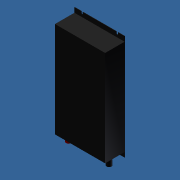
# Autodesk Inventor part: 2kW inverter
Saved by Autodesk Inventor 2012 (Build 160160000, 160)
## iProperties
Created: 2012-06-21
Part Number: 2kW inverter
Material: Default
Document SubType Name: Modeling
Designer: Ed
Density: 0.921071 g/cm^3
Mass: 5600 g
Surface Area: 2636.64 cm^2
Volume: 6079.88 cm^3
Author: Ed
Autodesk Inventor part; units mm, degrees
ref_plane "YZ Plane" through (0, 0, 0) normal (1, 0, 0) x (0, 1, 0)
ref_plane "XZ Plane" through (0, 0, 0) normal (0, 1, 0) x (-1, 0, 0)
ref_plane "XY Plane" through (0, 0, 0) normal (0, 0, 1) x (1, 0, 0)
sketch "Sketch1" plane through (0, 0, 0) normal (0, 0, 1) x (1, 0, 0)
  line L0 (-100.0125, -209.55) -> (100.0125, -209.55)
  line L1 (100.0125, -209.55) -> (100.0125, 209.55)
  line L2 (100.0125, 209.55) -> (-100.0125, 209.55)
  line L3 (-100.0125, 209.55) -> (-100.0125, -209.55)
  circle A0 centre (69.85, 203.2) radius 3.175
  line L4 (66.675, 209.55) -> (73.025, 209.55)
  line L5 (73.025, 209.55) -> (73.025, 203.2)
  line L6 (73.025, 203.2) -> (66.675, 203.2)
  line L7 (66.675, 203.2) -> (66.675, 209.55)
  line L8 (0, 209.55) -> (0, -209.55)
  line L9 (100.0125, 0) -> (-100.0125, 0)
  circle A1 centre (-69.85, 203.2) radius 3.175
  line L10 (-66.675, 209.55) -> (-73.025, 209.55)
  line L11 (-73.025, 209.55) -> (-73.025, 203.2)
  line L12 (-73.025, 203.2) -> (-66.675, 203.2)
  line L13 (-66.675, 203.2) -> (-66.675, 209.55)
  circle A2 centre (69.85, -203.2) radius 3.175
  line L14 (66.675, -209.55) -> (73.025, -209.55)
  line L15 (73.025, -209.55) -> (73.025, -203.2)
  line L16 (73.025, -203.2) -> (66.675, -203.2)
  line L17 (66.675, -203.2) -> (66.675, -209.55)
  circle A3 centre (-69.85, -203.2) radius 3.175
  line L18 (-66.675, -209.55) -> (-73.025, -209.55)
  line L19 (-73.025, -209.55) -> (-73.025, -203.2)
  line L20 (-73.025, -203.2) -> (-66.675, -203.2)
  line L21 (-66.675, -203.2) -> (-66.675, -209.55)
  point P0 (0, 0)
  point P1 (0, 0)
  dimension "d0" = 419.1
  dimension "d1" = 200.025
  dimension "d2" = 6.35
  dimension "d3" = 6.35
  dimension "d4" = 30.1625
  constraints: 44 end point, 18 symmetric about line, 8 point on circle, 6 midpoint, 5 coincident, 4 centre point, 4 parallel, 2 horizontal, 2 perpendicular, 1 point on line, 3 other
  measures "d0" distance of L2.end L0.start
  measures "d1" distance of L0.start L0.end
  measures "d2" diameter of A0
  measures "d3" distance of L4.end L5.end
  measures "d4" distance from line of L1 A0.centre
extrude "Extrusion1" add sketch "Sketch1" along normal blind 1.5875 contours L3 L9 L8 L0 L21 A3 L19 | L3 L2 L11 A1 L13 L8 L9 | L9 L1 L0 L15 A2 L17 L8 | L8 L2 L7 A0 L5 L1 L9
sketch "Sketch2" plane through (0, 0, 1.5875) normal (0, 0, 1) x (1, 0, 0)
  line L0 (100.0125, 209.55) -> (100.0125, -209.55) projected
  line L1 (-100.0125, -209.55) -> (-100.0125, 209.55) projected
  line L2 (-100.0125, 190.5) -> (100.0125, 190.5)
  line L3 (100.0125, 190.5) -> (100.0125, -190.5)
  line L4 (100.0125, -190.5) -> (-100.0125, -190.5)
  line L5 (-100.0125, -190.5) -> (-100.0125, 190.5)
  point P0 (0, 0)
  point P1 (-100.0125, 0)
  dimension "d7" = 381
  constraints: 8 end point, 2 midpoint, 2 parallel, 1 collinear, 1 horizontal, 1 perpendicular, 1 point on line
  measures "d7" distance between parallel lines of L4 L2
extrude "Extrusion2" add sketch "Sketch2" along normal blind 77.7875
sketch "Sketch3" plane through (-100.0125, -190.5, 1.5875) normal (0, -1, 0) x (1, 0, 0)
  line L0 (0, 0) -> (0, 77.7875) projected
  circle A0 centre (19.05, 42.8625) radius 9.525
  line L1 (0, -1.5875) -> (26.9875, -1.5875) projected
  point P0 (100.0125, -1.5875)
  dimension "d10" = 19.05
  dimension "d11" = 44.45
  dimension "d12" = 19.05
  constraints: 1 centre point
  measures "d10" diameter of A0
  measures "d11" distance from line of L1 A0.centre
  measures "d12" distance from line of A0.centre L0
extrude "Extrusion3" add sketch "Sketch3" along normal blind 33.3375
mirror "Mirror1" about plane through (0, 0, 0) normal (1, 0, 0) of "Extrusion3"
body "Solid1"
